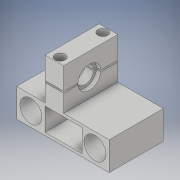
# Autodesk Inventor part: radiuscarrage
Saved by Autodesk Inventor 2019.1 (Build 231200000, 200)
## iProperties
Created: 2019-08-13
Part Number: radiuscarrage
Material: Generic
Document SubType Name: Modeling
Designer: Computus
Density: 1 g/cm^3
Appearance: Default
Author: Computus
## iProperties of the stored document radiuscarrage_3DPrint.ipt
Created: 2019-08-13
Part Number: radiuscarrage_3DPrint
Material: Generic
Document SubType Name: Modeling
Designer: Computus
Density: 1 g/cm^3
Appearance: Default
Author: Computus
Autodesk Inventor part; units mm, degrees
ref_plane "YZ Plane" through (0, 0, 0) normal (1, 0, 0) x (0, 1, 0)
ref_plane "XZ Plane" through (0, 0, 0) normal (0, 1, 0) x (-1, 0, 0)
sketch "Sketch1" plane through (0, 0, 0) normal (0, 1, 0) x (-1, 0, 0)
  line L0 (0, 0) -> (65, 0)
  line L1 (65, 0) -> (65, -38)
  line L2 (65, -38) -> (0, -38)
  line L3 (0, -38) -> (0, 0)
  dimension "d0" = 65
  dimension "d1" = 38
  constraints: 8 end point, 2 parallel, 1 horizontal, 1 perpendicular
  measures "d0" distance of L1.end L2.end
  measures "d1" distance of L0.end L1.end
extrude "Extrusion1" add sketch "Sketch1" along normal blind 20
sketch "Sketch2" plane through (-65, 0, 0) normal (0, 0, 1) x (1, 0, 0)
  circle A0 centre (10, 10) radius 7.75
  circle A1 centre (55, 10) radius 7.75
  line L0 (0, 0) -> (0, 20) projected
  line L1 (65, 0) -> (0, 0) projected
  dimension "d4" = 15.5
  dimension "d5" = 15.5
  dimension "d6" = 45
  dimension "d7" = 10
  dimension "d8" = 10
  dimension "d9" = 10
  constraints: 2 centre point
  measures "d4" diameter of A0
  measures "d5" diameter of A1
  measures "d6" distance of A1.centre A0.centre
  measures "d7" distance from line of A0.centre L0
  measures "d8" distance from line of L1 A0.centre
  measures "d9" distance from line of A1.centre L1
extrude "Extrusion2" cut sketch "Sketch2" against normal blind 60
sketch "Sketch3" plane through (-65, 0, 0) normal (0, 0, 1) x (1, 0, 0)
  line L0 (19.9566, 2) -> (45.9566, 2)
  line L1 (45.9566, 2) -> (45.9566, 18)
  line L2 (45.9566, 18) -> (19.9566, 18)
  line L3 (19.9566, 18) -> (19.9566, 2)
  line L4 (65, 0) -> (0, 0) projected
  dimension "d12" = 26
  dimension "d13" = 16
  dimension "d14" = 2
  constraints: 8 end point, 2 parallel, 1 horizontal, 1 perpendicular
  measures "d12" distance of L2.end L1.end
  measures "d13" distance of L1.end L0.end
  measures "d14" distance between parallel lines of L0 L4
extrude "Extrusion3" cut sketch "Sketch3" against normal blind 60
sketch "Sketch5" plane through (0, 20, 0) normal (0, 1, 0) x (1, 0, 0)
  line L0 (0, 38) -> (-65, 38) projected
  line L1 (-65, 0) -> (0, 0) projected
  line L2 (-45, 38) -> (-32, 38)
  line L3 (-32, 38) -> (-32, 0)
  line L4 (-32, 0) -> (-45, 0)
  line L5 (-45, 0) -> (-45, 38)
  line L6 (0, 0) -> (0, 38) projected
  dimension "d17" = 13
  dimension "d45" = 32
  constraints: 8 end point, 2 parallel, 1 horizontal, 1 perpendicular
  measures "d17" distance of L3.end L4.end
  measures "d45" distance between parallel lines of L6 L3
extrude "Extrusion4" add sketch "Sketch5" along normal blind 29 contours L3 L1 L5 L0
sketch "Sketch7" plane through (-65, 0, -38) normal (-1, 0, 0) x (0, 0, 1)
  circle A0 centre (20, 33) radius 6
  line L0 (0, 49) -> (38, 49) projected
  line L1 (0, 0) -> (0, 20) projected
  point P0 (38, 0)
  point P1 (0, 46)
  dimension "d20" = 12
  dimension "d21" = 16
  dimension "d22" = 20
  constraints: 1 centre point, 1 other
  measures "d20" diameter of A0
  measures "d22" distance from line of L1 A0.centre
extrude "Extrusion5" cut sketch "Sketch7" along normal mid plane 600
ref_plane "Work Plane1" through (0, 33, 0) normal (0, 1, 0) x (1, 0, 0)
sketch "Sketch10" plane through (0, 33, 0) normal (0, 1, 0) x (1, 0, 0)
  line L0 (-45.6413, -0.955) -> (-31.8263, -0.955)
  line L1 (-31.8263, -0.955) -> (-31.8263, 38.7188)
  line L2 (-31.8263, 38.7188) -> (-45.6413, 38.7188)
  line L3 (-45.6413, 38.7188) -> (-45.6413, -0.955)
  point P0 (0, 0)
  constraints: 8 end point, 2 parallel, 1 horizontal, 1 perpendicular
sketch "Sketch11" plane through (0, 49, 0) normal (0, 1, 0) x (1, 0, 0)
  circle A0 centre (-38.5, 4) radius 1.5
  circle A1 centre (-38.5, 34) radius 1.5
  line L0 (-45, 0) -> (-32, 0) projected
  line L1 (-45, 38) -> (-45, 0) projected
  point P0 (0, 0)
  point P1 (-65, 38)
  dimension "d33" = 3
  dimension "d34" = 3
  dimension "d35" = 30
  dimension "d36" = 4
  dimension "d37" = 6.5
  dimension "d38" = 6.5
  constraints: 2 centre point, 1 other
  measures "d33" diameter of A0
  measures "d34" diameter of A1
  measures "d35" distance of A1.centre A0.centre
  measures "d36" distance from line of L0 A0.centre
extrude "Extrusion9" cut sketch "Sketch11" against normal blind 27
sketch "Sketch12" plane through (0, 49, 0) normal (0, 1, 0) x (1, 0, 0)
  circle A0 centre (-38.5, 34) radius 1.5 projected
  circle A1 centre (-38.5, 34) radius 3.5
  circle A2 centre (-38.5, 4) radius 1.5 projected
  circle A3 centre (-38.5, 4) radius 1.5
  circle A4 centre (-38.5, 4) radius 3.5
  point P0 (0, 0)
  dimension "d42" = 7
  dimension "d55" = 7
  constraints: 3 centre point, 3 coincident
  measures "d42" diameter of A1
  measures "d55" diameter of A4
sketch "Sketch13" plane through (-45, 20, -38) normal (-1, 0, 0) x (0, 0, 1)
  circle A0 centre (20, 13) radius 6 projected
  circle A1 centre (20, 13) radius 6
  circle A2 centre (20, 13) radius 8
  point P0 (38, -20)
  dimension "d46" = 16
  constraints: 2 centre point, 2 coincident
  measures "d46" diameter of A2
extrude "Extrusion11" cut sketch "Sketch13" against normal blind 4
sketch "Sketch14" plane through (-32, 20, 0) normal (1, 0, 0) x (0, 0, -1)
  circle A0 centre (18, 13) radius 6 projected
  circle A1 centre (18, 13) radius 6
  circle A2 centre (18, 13) radius 8
  point P0 (0, -20)
  dimension "d49" = 16
  constraints: 2 centre point, 2 coincident
  measures "d49" diameter of A2
extrude "Extrusion12" cut sketch "Sketch14" against normal blind 3
extrude "Extrusion13" cut sketch "Sketch10" along normal mid plane 1
extrude "Extrusion14" cut sketch "Sketch12" against normal blind 13
body "Solid1"
